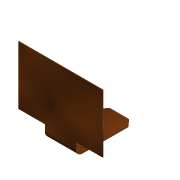
# Autodesk Inventor part: ECoG64Ch
Saved by Autodesk Inventor 2014 (Build 180170000, 170)
## iProperties
Created: 2016-07-07
Part Number: ECoG64Ch
Material: Generic
Document SubType Name: Modeling
Designer: Camilo
Density: 1 g/cm^3
Appearance: Brown
Author: Camilo
Autodesk Inventor part; units mm, degrees
note: some values were not read from the file. Chosen so that the rebuilt part matches the saved one: bend side of "Bend Part1".
ref_plane "YZ Plane" through (0, 0, 0) normal (1, 0, 0) x (0, 1, 0)
ref_plane "XZ Plane" through (0, 0, 0) normal (0, 1, 0) x (-1, 0, 0)
ref_plane "XY Plane" through (0, 0, 0) normal (0, 0, 1) x (1, 0, 0)
sketch "Sketch1" plane through (0, 0, 0) normal (0, 1, 0) x (-1, 0, 0)
  line L0 (-6.425, -4.45) -> (6.425, -4.45)
  line L1 (6.425, -4.45) -> (6.425, 4.45)
  line L2 (6.425, 4.45) -> (-6.425, 4.45)
  line L3 (-6.425, 4.45) -> (-6.425, -4.45)
  line L4 (-6.425, -4.45) -> (6.425, 4.45) construction
  line L5 (6.425, -4.45) -> (-6.425, 4.45) construction
  line L6 (-2.3625, -4.45) -> (2.3625, -4.45)
  line L7 (2.3625, -4.45) -> (2.3625, -14)
  line L8 (-2.3625, -14) -> (-2.3625, -4.45)
  line L9 (1.45, -15.01) -> (-1.45, -15.01)
  line L10 (2.3625, -14) -> (1.45, -15.01)
  line L11 (-1.45, -15.01) -> (-2.3625, -14)
  constraints: 24 end point, 2 point on line
extrude "Extrusion1" add sketch "Sketch1" along normal blind 0.1
sketch "Sketch2" plane through (0, 0, 0) normal (0, -1, 0) x (1, 0, 0)
  line L0 (-2.3625, -4.45) -> (2.3625, -4.45)
  line L1 (-2.3625, -5.45) -> (2.3625, -5.45)
  point P0 (0, 0)
  dimension "d2" = 1
  constraints: 4 end point, 1 parallel
  measures "d2" distance between parallel lines of L1 L0
bend part "Bend Part1" radius 1 angle 90 line through (-2.3625, 0, -4.45) along (1, 0, 0) centre toward (0, 1, 0) moving side (0, 0, -1) both sides no
body "Solid1"
